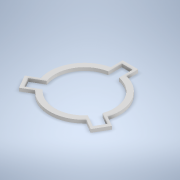
# Autodesk Inventor part: 로드셀 부품1
Saved by Autodesk Inventor 2021 (Build 250183000, 183)
## iProperties
Created: 2021-08-23
Part Number: 로드셀 부품1
Material: 일반
Document SubType Name: Modeling
Designer: Dongyoon
Density: 1 g/cm^3
Appearance: 기본값
Author: Dongyoon
Autodesk Inventor part; units mm, degrees
ref_plane "YZ Plane" through (0, 0, 0) normal (1, 0, 0) x (0, 1, 0)
ref_plane "XZ Plane" through (0, 0, 0) normal (0, 1, 0) x (-1, 0, 0)
ref_plane "XY Plane" through (0, 0, 0) normal (0, 0, 1) x (1, 0, 0)
sketch "스케치1" plane through (0, 0, 0) normal (0, 1, 0) x (-1, 0, 0)
  arc A0 (3.6, -15.8462) -> (-3.6, -15.8462) centre (0, 0) ccw
  arc A1 (2.5, -13.5208) -> (-2.5, -13.5208) centre (0, 0) ccw
  line L0 (3.6, -15.8462) -> (3.6, -21.3462)
  line L1 (3.6, -21.3462) -> (-3.6, -21.3462)
  line L2 (-3.6, -21.3462) -> (-3.6, -15.8462)
  line L3 (2.5, -19.8462) -> (-2.5, -19.8462)
  line L4 (-2.5, -19.8462) -> (-2.5, -13.5208)
  line L5 (2.5, -13.5208) -> (2.5, -19.8462)
  arc A2 (11.9232, 11.0408) -> (15.5232, 4.8054) centre (0, 0) ccw
  arc A3 (10.4594, 8.9255) -> (12.9594, 4.5953) centre (0, 0) ccw
  line L6 (11.9232, 11.0408) -> (16.6864, 13.7908)
  line L7 (16.6864, 13.7908) -> (20.2864, 7.5554)
  line L8 (20.2864, 7.5554) -> (15.5232, 4.8054)
  line L9 (15.9373, 12.0882) -> (18.4373, 7.758)
  line L10 (18.4373, 7.758) -> (12.9594, 4.5953)
  line L11 (10.4594, 8.9255) -> (15.9373, 12.0882)
  arc A4 (-15.5232, 4.8054) -> (-11.9232, 11.0408) centre (0, 0) ccw
  arc A5 (-12.9594, 4.5953) -> (-10.4594, 8.9255) centre (0, 0) ccw
  line L12 (-15.5232, 4.8054) -> (-20.2864, 7.5554)
  line L13 (-20.2864, 7.5554) -> (-16.6864, 13.7908)
  line L14 (-16.6864, 13.7908) -> (-11.9232, 11.0408)
  line L15 (-18.4373, 7.758) -> (-15.9373, 12.0882)
  line L16 (-15.9373, 12.0882) -> (-10.4594, 8.9255)
  line L17 (-12.9594, 4.5953) -> (-18.4373, 7.758)
  point P0 (-12.9594, 4.5953)
  point P1 (10.4594, 8.9255)
  point P2 (15.5232, 4.8054)
  point P3 (11.9232, 11.0408)
  point P4 (-11.9232, 11.0408)
  point P5 (-15.5232, 4.8054)
  dimension "d0" = 32.5
  dimension "d1" = 2.5
  dimension "d2" = 5.5
  dimension "d3" = 5.5
  dimension "d4" = 7.2
  dimension "d5" = 1.5
  dimension "d6" = 5
  dimension "d7" = 1.1
  dimension "d10" = 360
  constraints: 36 end point, 12 point on circle, 6 centre point, 4 coincident, 3 perpendicular, 1 horizontal, 1 parallel, 1 vertical, 55 other
  measures "d0" diameter of A0
  measures "d1" radial gap between concentric circles of A1 A0
  measures "d2" distance of L0.start L0.end
  measures "d3" distance of L2.end L1.end
  measures "d4" distance of L0.end L1.end
  measures "d5" distance between parallel lines of L1 L3
  measures "d6" distance of L3.start L3.end
  measures "d7" distance between parallel lines of L2 L4
extrude "돌출1" add sketch "스케치1" along normal blind 1.5 contours A2 L5 A1 L10 A0 | L0 L1 L2 A2 L4 L3 L5 | A0 L10 L9 L11 L6 L7 L8 | A2 A0 L17 A1 L4 | L11 A1 L16 A0 | L12 L13 L14 A0 L16 L15 L17
